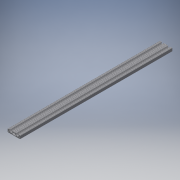
# Autodesk Inventor part: 24in_2012
Saved by Autodesk Inventor 2019 (Build 230136000, 136)
## iProperties
Company: 80/20 Inc.
Created: 2014-04-23
Part Number: 24in_2012
Material: Generic
Document SubType Name: Modeling
Density: 1 g/cm^3
Vendor: 80/20 Inc.
Engineer: Ross Bowman
Designer: Ross Bowman
Catalog Web Link: 8020.net
Appearance: Default
Material: 6105-T5 Aluminum
Author: Ross Bowman
Keywords: 80/20 , 8020 , T-Slot , Extrusion
Autodesk Inventor part; units mm, degrees
ref_plane "YZ Plane" through (0, 0, 0) normal (1, 0, 0) x (0, 1, 0)
ref_plane "XZ Plane" through (0, 0, 0) normal (0, 1, 0) x (-1, 0, 0)
ref_plane "XY Plane" through (0, 0, 0) normal (0, 0, 1) x (1, 0, 0)
sketch "Sketch1" plane through (0, 0, 0) normal (0, 0, 1) x (1, 0, 0)
  arc A0 (-8.2061, -3.1475) -> (-7.8618, -4.0207) centre (-7.8531, -3.5128) ccw
  line L0 (-0.8184, 3.9914) -> (-8.2061, -3.1475)
  arc A1 (-0.4592, 4.1402) -> (-0.8184, 3.9914) centre (-0.4592, 3.6322) ccw
  line L1 (0.4145, 4.1402) -> (-0.4592, 4.1402)
  arc A2 (0.8488, 3.962) -> (0.4145, 4.1402) centre (0.4606, 3.6343) ccw
  line L2 (8.2061, -3.1475) -> (0.8488, 3.962)
  arc A3 (7.8618, -4.0207) -> (8.2061, -3.1475) centre (7.8531, -3.5128) ccw
  line L3 (-7.8618, -4.0207) -> (7.8618, -4.0207)
  circle A4 centre (21.4376, -2.3876) radius 2.032
  circle A5 centre (-21.4376, -2.3876) radius 2.032
  arc A6 (16.9463, 6.35) -> (15.8972, 5.301) centre (16.9463, 5.301) ccw
  line L4 (15.8972, 5.301) -> (15.8972, 5.1892)
  arc A7 (15.8972, 5.1892) -> (16.9463, 4.1402) centre (16.9463, 5.1892) ccw
  line L5 (16.9463, 4.1402) -> (19.0952, 4.1402)
  arc A8 (19.8159, 2.3571) -> (19.0952, 4.1402) centre (19.0952, 3.103) ccw
  line L6 (19.8159, 2.3571) -> (16.5346, -0.8136)
  arc A9 (14.3374, -1.7018) -> (16.5346, -0.8136) centre (14.3374, 1.4602) ccw
  line L7 (14.3374, -1.7018) -> (11.0626, -1.7018)
  arc A10 (8.8654, -0.8136) -> (11.0626, -1.7018) centre (11.0626, 1.4602) ccw
  line L8 (8.8654, -0.8136) -> (5.5841, 2.3571)
  arc A11 (6.3048, 4.1402) -> (5.5841, 2.3571) centre (6.3048, 3.103) ccw
  line L9 (6.3048, 4.1402) -> (8.4349, 4.1402)
  arc A12 (8.4349, 4.1402) -> (9.4839, 5.1892) centre (8.4349, 5.1892) ccw
  line L10 (9.4839, 5.1892) -> (9.4839, 5.301)
  arc A13 (9.4839, 5.301) -> (8.4349, 6.35) centre (8.4349, 5.301) ccw
  line L11 (8.4349, 6.35) -> (7.3479, 6.35)
  arc A14 (6.332, 6.35) -> (7.3479, 6.35) centre (6.8399, 6.3541) ccw
  line L12 (6.332, 6.35) -> (3.1719, 6.35)
  arc A15 (2.156, 6.35) -> (3.1719, 6.35) centre (2.6639, 6.3541) ccw
  line L13 (2.156, 6.35) -> (-2.156, 6.35)
  arc A16 (-3.1719, 6.35) -> (-2.156, 6.35) centre (-2.6639, 6.3541) ccw
  line L14 (-3.1719, 6.35) -> (-6.3893, 6.35)
  arc A17 (-7.4052, 6.35) -> (-6.3893, 6.35) centre (-6.8973, 6.3541) ccw
  line L15 (-7.4052, 6.35) -> (-8.4349, 6.35)
  arc A18 (-8.4349, 6.35) -> (-9.4839, 5.301) centre (-8.4349, 5.301) ccw
  line L16 (-9.4839, 5.301) -> (-9.4839, 5.1892)
  arc A19 (-9.4839, 5.1892) -> (-8.4349, 4.1402) centre (-8.4349, 5.1892) ccw
  line L17 (-8.4349, 4.1402) -> (-6.3048, 4.1402)
  arc A20 (-5.5841, 2.3571) -> (-6.3048, 4.1402) centre (-6.3048, 3.103) ccw
  line L18 (-5.5841, 2.3571) -> (-8.8654, -0.8136)
  arc A21 (-11.0626, -1.7018) -> (-8.8654, -0.8136) centre (-11.0626, 1.4602) ccw
  line L19 (-11.0626, -1.7018) -> (-14.3374, -1.7018)
  arc A22 (-16.5346, -0.8136) -> (-14.3374, -1.7018) centre (-14.3374, 1.4602) ccw
  line L20 (-16.5346, -0.8136) -> (-19.809, 2.3504)
  arc A23 (-19.0855, 4.1402) -> (-19.809, 2.3504) centre (-19.0855, 3.0991) ccw
  line L21 (-19.0855, 4.1402) -> (-17.0099, 4.1402)
  arc A24 (-17.0099, 4.1402) -> (-15.9609, 5.1892) centre (-17.0099, 5.1892) ccw
  line L22 (-15.9609, 5.1892) -> (-15.9609, 5.301)
  arc A25 (-15.9609, 5.301) -> (-17.0099, 6.35) centre (-17.0099, 5.301) ccw
  line L23 (-17.0099, 6.35) -> (-18.0395, 6.35)
  arc A26 (-19.0555, 6.35) -> (-18.0395, 6.35) centre (-18.5475, 6.3541) ccw
  line L24 (-19.0555, 6.35) -> (-22.2504, 6.35)
  arc A27 (-23.2664, 6.354) -> (-22.2504, 6.35) centre (-22.7584, 6.3541) ccw
  arc A28 (-23.2664, 6.354) -> (-25.4, 4.2459) centre (-23.2918, 4.2459) ccw
  line L25 (-25.4, 4.2459) -> (-25.4, -4.2459)
  arc A29 (-25.4, -4.2459) -> (-23.2881, -6.4371) centre (-23.2933, -4.3288) ccw
  arc A30 (-22.2765, -6.35) -> (-23.2881, -6.4371) centre (-22.7808, -6.4114) ccw
  line L26 (-22.2765, -6.35) -> (-19.0448, -6.35)
  arc A31 (-18.0363, -6.35) -> (-19.0448, -6.35) centre (-18.5406, -6.4114) ccw
  line L27 (-18.0363, -6.35) -> (-7.4084, -6.35)
  arc A32 (-6.3999, -6.35) -> (-7.4084, -6.35) centre (-6.9041, -6.4114) ccw
  line L28 (-6.3999, -6.35) -> (-3.1684, -6.35)
  arc A33 (-2.1599, -6.35) -> (-3.1684, -6.35) centre (-2.6641, -6.4114) ccw
  line L29 (-2.1599, -6.35) -> (2.1135, -6.35)
  arc A34 (3.122, -6.35) -> (2.1135, -6.35) centre (2.6177, -6.4114) ccw
  line L30 (3.122, -6.35) -> (6.3882, -6.35)
  arc A35 (7.3967, -6.35) -> (6.3882, -6.35) centre (6.8925, -6.4114) ccw
  line L31 (7.3967, -6.35) -> (18.0231, -6.35)
  arc A36 (19.0317, -6.35) -> (18.0231, -6.35) centre (18.5274, -6.4114) ccw
  line L32 (19.0317, -6.35) -> (22.2866, -6.35)
  arc A37 (23.2982, -6.4371) -> (22.2866, -6.35) centre (22.7909, -6.4114) ccw
  arc A38 (23.2982, -6.4371) -> (25.4, -4.2459) centre (23.2933, -4.3288) ccw
  line L33 (25.4, -4.2459) -> (25.4, 4.2355)
  arc A39 (25.4, 4.2355) -> (23.2665, 6.354) centre (23.2918, 4.2459) ccw
  arc A40 (22.2505, 6.35) -> (23.2665, 6.354) centre (22.7585, 6.3541) ccw
  line L34 (22.2505, 6.35) -> (18.998, 6.35)
  arc A41 (17.9823, 6.35) -> (18.998, 6.35) centre (18.4902, 6.3374) ccw
  line L35 (17.9823, 6.35) -> (16.9463, 6.35)
  point P0 (0, 0)
  constraints: 80 point on circle, 72 end point, 42 centre point
extrude "Extrusion1" add sketch "Sketch1" against normal blind 609.6
body "Solid1"
